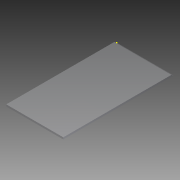
# Autodesk Inventor part: teto02
Saved by Autodesk Inventor 2015 (Build 190159000, 159)
## iProperties
Created: 2016-08-07
Part Number: teto02
Material: Polycarbonate, Clear
Document SubType Name: Modeling
Designer: Gabriel
Density: 1.2 g/cm^3
Appearance: Polycarbonate - Clear
Author: Gabriel
Autodesk Inventor part; units mm, degrees
ref_plane "YZ Plane" through (0, 0, 0) normal (1, 0, 0) x (0, 1, 0)
ref_plane "XZ Plane" through (0, 0, 0) normal (0, 1, 0) x (-1, 0, 0)
ref_plane "XY Plane" through (0, 0, 0) normal (0, 0, 1) x (1, 0, 0)
sketch "Sketch1" plane through (0, 0, 0) normal (0, 0, 1) x (1, 0, 0)
  point P0 (0, 0)
sketch "Sketch2" plane through (0, 0, 0) normal (0, 0, 1) x (1, 0, 0)
  line L0 (0, 0) -> (219, 0)
  line L1 (219, 0) -> (219, 7)
  line L2 (219, 7) -> (0, 7)
  line L3 (0, 7) -> (0, 0)
  dimension "d0" = 219
  dimension "d1" = 7
  constraints: 8 end point, 2 parallel, 1 horizontal, 1 perpendicular
  measures "d0" distance of L2.end L1.end
  measures "d1" distance of L1.end L0.end
extrude "Extrusion1" add sketch "Sketch2" along normal blind 424
sketch "Sketch3" plane through (219, 7, 424) normal (1, 0, 0) x (0, 0, -1)
  line L0 (424, -7) -> (431.4138, -7)
  line L1 (424, -7) -> (430.4406, -11.8059)
  line L2 (424, -7) -> (432.0361, -7) construction
  line L3 (424, -7) -> (414.619, 0)
  line L4 (424, 0) -> (0, 0) projected
  line L5 (414.619, 0) -> (424, 0)
  line L6 (424, -7) -> (424, 0)
  line L7 (424, -7) -> (424, 0) projected
  line L8 (424, 0) -> (424, -7)
  dimension "d4" = 36.73
  constraints: 14 end point, 2 collinear, 2 horizontal, 1 equal length, 1 perpendicular, 1 point on line
  measures "d4" angle of L1 L2
extrude "Extrusion2" cut sketch "Sketch3" against normal blind 334.4875
body "Solid1"
